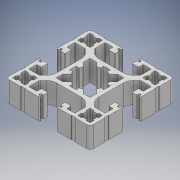
# Autodesk Inventor part: PERFIL_ESTRUTURAL_40X40_EIXO_Y_PERPENDICULAR
Saved by Autodesk Inventor 2018 (Build 220112000, 112)
## iProperties
Created: 2018-10-11
Part Number: PERFIL_ESTRUTURAL_40X40_EIXO_Y_PERPENDICULAR
Material: Genérico
Document SubType Name: Modeling
Designer: Usuario
Density: 1 g/cm^3
Appearance: Padrão
Author: Usuario
Autodesk Inventor part; units mm, degrees
ref_plane "YZ Plane" through (0, 0, 0) normal (1, 0, 0) x (0, 1, 0)
ref_plane "XZ Plane" through (0, 0, 0) normal (0, 1, 0) x (-1, 0, 0)
ref_plane "XY Plane" through (0, 0, 0) normal (0, 0, 1) x (1, 0, 0)
sketch "Esboço1" plane through (0, 0, 0) normal (0, 0, 1) x (1, 0, 0)
  arc A0 (-10, 5.8076) -> (-11.4645, 9.3431) centre (-15, 5.8076) ccw
  line L0 (-10, -5.8076) -> (-10, 5.8076)
  arc A1 (-11.4645, -9.3431) -> (-10, -5.8076) centre (-15, -5.8076) ccw
  line L1 (-12.8284, -10.7071) -> (-11.4645, -9.3431)
  arc A2 (-13.5355, -11) -> (-12.8284, -10.7071) centre (-13.5355, -10) ccw
  line L2 (-17.9, -11) -> (-13.5355, -11)
  arc A3 (-18.2, -10.7) -> (-17.9, -11) centre (-17.9, -10.7) ccw
  line L3 (-18.2, -7.45) -> (-18.2, -10.7)
  arc A4 (-17.9, -7.15) -> (-18.2, -7.45) centre (-17.9, -7.45) ccw
  line L4 (-16.3, -7.15) -> (-17.9, -7.15)
  arc A5 (-16.3, -7.15) -> (-16, -6.85) centre (-16.3, -6.85) ccw
  line L5 (-16, -4.4) -> (-16, -6.85)
  arc A6 (-16, -4.4) -> (-16.3, -4.1) centre (-16.3, -4.4) ccw
  line L6 (-17.9, -4.1) -> (-16.3, -4.1)
  arc A7 (-17.9, -4.1) -> (-18.2, -4.4) centre (-17.9, -4.4) ccw
  line L7 (-18.2, -5.05) -> (-18.2, -4.4)
  arc A8 (-18.5, -5.35) -> (-18.2, -5.05) centre (-18.5, -5.05) ccw
  line L8 (-18.9, -5.35) -> (-18.5, -5.35)
  arc A9 (-19.2, -5.05) -> (-18.9, -5.35) centre (-18.9, -5.05) ccw
  line L9 (-19.2, -4.4) -> (-19.2, -5.05)
  arc A10 (-19.2, -4.4) -> (-19.5, -4.1) centre (-19.5, -4.4) ccw
  line L10 (-19.7, -4.1) -> (-19.5, -4.1)
  arc A11 (-19.7, -4.1) -> (-20, -4.4) centre (-19.7, -4.4) ccw
  line L11 (-20, -11) -> (-20, -4.4)
  line L12 (-19.75, -11) -> (-20, -11)
  line L13 (-19.75, -13) -> (-19.75, -11)
  line L14 (-20, -13) -> (-19.75, -13)
  line L15 (-20, -18.5) -> (-20, -13)
  arc A12 (-20, -18.5) -> (-18.5, -20) centre (-18.5, -18.5) ccw
  line L16 (-13, -20) -> (-18.5, -20)
  line L17 (-13, -19.75) -> (-13, -20)
  line L18 (-11, -19.75) -> (-13, -19.75)
  line L19 (-11, -20) -> (-11, -19.75)
  line L20 (-4.4, -20) -> (-11, -20)
  arc A13 (-4.4, -20) -> (-4.1, -19.7) centre (-4.4, -19.7) ccw
  line L21 (-4.1, -19.5) -> (-4.1, -19.7)
  arc A14 (-4.1, -19.5) -> (-4.4, -19.2) centre (-4.4, -19.5) ccw
  line L22 (-5.05, -19.2) -> (-4.4, -19.2)
  arc A15 (-5.35, -18.9) -> (-5.05, -19.2) centre (-5.05, -18.9) ccw
  line L23 (-5.35, -18.5) -> (-5.35, -18.9)
  arc A16 (-5.05, -18.2) -> (-5.35, -18.5) centre (-5.05, -18.5) ccw
  line L24 (-4.4, -18.2) -> (-5.05, -18.2)
  arc A17 (-4.4, -18.2) -> (-4.1, -17.9) centre (-4.4, -17.9) ccw
  line L25 (-4.1, -16.3) -> (-4.1, -17.9)
  arc A18 (-4.1, -16.3) -> (-4.4, -16) centre (-4.4, -16.3) ccw
  line L26 (-6.85, -16) -> (-4.4, -16)
  arc A19 (-6.85, -16) -> (-7.15, -16.3) centre (-6.85, -16.3) ccw
  line L27 (-7.15, -17.9) -> (-7.15, -16.3)
  arc A20 (-7.45, -18.2) -> (-7.15, -17.9) centre (-7.45, -17.9) ccw
  line L28 (-10.7, -18.2) -> (-7.45, -18.2)
  arc A21 (-11, -17.9) -> (-10.7, -18.2) centre (-10.7, -17.9) ccw
  line L29 (-11, -13.5355) -> (-11, -17.9)
  arc A22 (-10.7071, -12.8284) -> (-11, -13.5355) centre (-10, -13.5355) ccw
  line L30 (-9.3431, -11.4645) -> (-10.7071, -12.8284)
  arc A23 (-5.8076, -10) -> (-9.3431, -11.4645) centre (-5.8076, -15) ccw
  line L31 (5.8076, -10) -> (-5.8076, -10)
  arc A24 (9.3431, -11.4645) -> (5.8076, -10) centre (5.8076, -15) ccw
  line L32 (10.7071, -12.8284) -> (9.3431, -11.4645)
  arc A25 (11, -13.5355) -> (10.7071, -12.8284) centre (10, -13.5355) ccw
  line L33 (11, -17.9) -> (11, -13.5355)
  arc A26 (10.7, -18.2) -> (11, -17.9) centre (10.7, -17.9) ccw
  line L34 (7.45, -18.2) -> (10.7, -18.2)
  arc A27 (7.15, -17.9) -> (7.45, -18.2) centre (7.45, -17.9) ccw
  line L35 (7.15, -16.3) -> (7.15, -17.9)
  arc A28 (7.15, -16.3) -> (6.85, -16) centre (6.85, -16.3) ccw
  line L36 (4.4, -16) -> (6.85, -16)
  arc A29 (4.4, -16) -> (4.1, -16.3) centre (4.4, -16.3) ccw
  line L37 (4.1, -17.9) -> (4.1, -16.3)
  arc A30 (4.1, -17.9) -> (4.4, -18.2) centre (4.4, -17.9) ccw
  line L38 (5.05, -18.2) -> (4.4, -18.2)
  arc A31 (5.35, -18.5) -> (5.05, -18.2) centre (5.05, -18.5) ccw
  line L39 (5.35, -18.9) -> (5.35, -18.5)
  arc A32 (5.05, -19.2) -> (5.35, -18.9) centre (5.05, -18.9) ccw
  line L40 (4.4, -19.2) -> (5.05, -19.2)
  arc A33 (4.4, -19.2) -> (4.1, -19.5) centre (4.4, -19.5) ccw
  line L41 (4.1, -19.7) -> (4.1, -19.5)
  arc A34 (4.1, -19.7) -> (4.4, -20) centre (4.4, -19.7) ccw
  line L42 (11, -20) -> (4.4, -20)
  line L43 (11, -19.75) -> (11, -20)
  line L44 (13, -19.75) -> (11, -19.75)
  line L45 (13, -20) -> (13, -19.75)
  line L46 (18.5, -20) -> (13, -20)
  arc A35 (18.5, -20) -> (20, -18.5) centre (18.5, -18.5) ccw
  line L47 (20, -13) -> (20, -18.5)
  line L48 (19.75, -13) -> (20, -13)
  line L49 (19.75, -11) -> (19.75, -13)
  line L50 (20, -11) -> (19.75, -11)
  line L51 (20, -4.4) -> (20, -11)
  arc A36 (20, -4.4) -> (19.7, -4.1) centre (19.7, -4.4) ccw
  line L52 (19.5, -4.1) -> (19.7, -4.1)
  arc A37 (19.5, -4.1) -> (19.2, -4.4) centre (19.5, -4.4) ccw
  line L53 (19.2, -5.05) -> (19.2, -4.4)
  arc A38 (18.9, -5.35) -> (19.2, -5.05) centre (18.9, -5.05) ccw
  line L54 (18.5, -5.35) -> (18.9, -5.35)
  arc A39 (18.2, -5.05) -> (18.5, -5.35) centre (18.5, -5.05) ccw
  line L55 (18.2, -4.4) -> (18.2, -5.05)
  arc A40 (18.2, -4.4) -> (17.9, -4.1) centre (17.9, -4.4) ccw
  line L56 (16.3, -4.1) -> (17.9, -4.1)
  arc A41 (16.3, -4.1) -> (16, -4.4) centre (16.3, -4.4) ccw
  line L57 (16, -6.85) -> (16, -4.4)
  arc A42 (16, -6.85) -> (16.3, -7.15) centre (16.3, -6.85) ccw
  line L58 (17.9, -7.15) -> (16.3, -7.15)
  arc A43 (18.2, -7.45) -> (17.9, -7.15) centre (17.9, -7.45) ccw
  line L59 (18.2, -10.7) -> (18.2, -7.45)
  arc A44 (17.9, -11) -> (18.2, -10.7) centre (17.9, -10.7) ccw
  line L60 (13.5355, -11) -> (17.9, -11)
  arc A45 (12.8284, -10.7071) -> (13.5355, -11) centre (13.5355, -10) ccw
  line L61 (11.4645, -9.3431) -> (12.8284, -10.7071)
  arc A46 (10, -5.8076) -> (11.4645, -9.3431) centre (15, -5.8076) ccw
  line L62 (10, 5.8076) -> (10, -5.8076)
  arc A47 (11.4645, 9.3431) -> (10, 5.8076) centre (15, 5.8076) ccw
  line L63 (12.8284, 10.7071) -> (11.4645, 9.3431)
  arc A48 (13.5355, 11) -> (12.8284, 10.7071) centre (13.5355, 10) ccw
  line L64 (17.9, 11) -> (13.5355, 11)
  arc A49 (18.2, 10.7) -> (17.9, 11) centre (17.9, 10.7) ccw
  line L65 (18.2, 7.45) -> (18.2, 10.7)
  arc A50 (17.9, 7.15) -> (18.2, 7.45) centre (17.9, 7.45) ccw
  line L66 (16.3, 7.15) -> (17.9, 7.15)
  arc A51 (16.3, 7.15) -> (16, 6.85) centre (16.3, 6.85) ccw
  line L67 (16, 4.4) -> (16, 6.85)
  arc A52 (16, 4.4) -> (16.3, 4.1) centre (16.3, 4.4) ccw
  line L68 (17.9, 4.1) -> (16.3, 4.1)
  arc A53 (17.9, 4.1) -> (18.2, 4.4) centre (17.9, 4.4) ccw
  line L69 (18.2, 5.05) -> (18.2, 4.4)
  arc A54 (18.5, 5.35) -> (18.2, 5.05) centre (18.5, 5.05) ccw
  line L70 (18.9, 5.35) -> (18.5, 5.35)
  arc A55 (19.2, 5.05) -> (18.9, 5.35) centre (18.9, 5.05) ccw
  line L71 (19.2, 4.4) -> (19.2, 5.05)
  arc A56 (19.2, 4.4) -> (19.5, 4.1) centre (19.5, 4.4) ccw
  line L72 (19.7, 4.1) -> (19.5, 4.1)
  arc A57 (19.7, 4.1) -> (20, 4.4) centre (19.7, 4.4) ccw
  line L73 (20, 11) -> (20, 4.4)
  line L74 (19.75, 11) -> (20, 11)
  line L75 (19.75, 13) -> (19.75, 11)
  line L76 (20, 13) -> (19.75, 13)
  line L77 (20, 18.5) -> (20, 13)
  arc A58 (20, 18.5) -> (18.5, 20) centre (18.5, 18.5) ccw
  line L78 (13, 20) -> (18.5, 20)
  line L79 (13, 19.75) -> (13, 20)
  line L80 (11, 19.75) -> (13, 19.75)
  line L81 (11, 20) -> (11, 19.75)
  line L82 (4.4, 20) -> (11, 20)
  arc A59 (4.4, 20) -> (4.1, 19.7) centre (4.4, 19.7) ccw
  line L83 (4.1, 19.5) -> (4.1, 19.7)
  arc A60 (4.1, 19.5) -> (4.4, 19.2) centre (4.4, 19.5) ccw
  line L84 (5.05, 19.2) -> (4.4, 19.2)
  arc A61 (5.35, 18.9) -> (5.05, 19.2) centre (5.05, 18.9) ccw
  line L85 (5.35, 18.5) -> (5.35, 18.9)
  arc A62 (5.05, 18.2) -> (5.35, 18.5) centre (5.05, 18.5) ccw
  line L86 (4.4, 18.2) -> (5.05, 18.2)
  arc A63 (4.4, 18.2) -> (4.1, 17.9) centre (4.4, 17.9) ccw
  line L87 (4.1, 16.3) -> (4.1, 17.9)
  arc A64 (4.1, 16.3) -> (4.4, 16) centre (4.4, 16.3) ccw
  line L88 (6.85, 16) -> (4.4, 16)
  arc A65 (6.85, 16) -> (7.15, 16.3) centre (6.85, 16.3) ccw
  line L89 (7.15, 17.9) -> (7.15, 16.3)
  arc A66 (7.45, 18.2) -> (7.15, 17.9) centre (7.45, 17.9) ccw
  line L90 (10.7, 18.2) -> (7.45, 18.2)
  arc A67 (11, 17.9) -> (10.7, 18.2) centre (10.7, 17.9) ccw
  line L91 (11, 13.5355) -> (11, 17.9)
  arc A68 (10.7071, 12.8284) -> (11, 13.5355) centre (10, 13.5355) ccw
  line L92 (9.3431, 11.4645) -> (10.7071, 12.8284)
  arc A69 (5.8076, 10) -> (9.3431, 11.4645) centre (5.8076, 15) ccw
  line L93 (-5.8076, 10) -> (5.8076, 10)
  arc A70 (-9.3431, 11.4645) -> (-5.8076, 10) centre (-5.8076, 15) ccw
  line L94 (-10.7071, 12.8284) -> (-9.3431, 11.4645)
  arc A71 (-11, 13.5355) -> (-10.7071, 12.8284) centre (-10, 13.5355) ccw
  line L95 (-11, 17.9) -> (-11, 13.5355)
  arc A72 (-10.7, 18.2) -> (-11, 17.9) centre (-10.7, 17.9) ccw
  line L96 (-7.45, 18.2) -> (-10.7, 18.2)
  arc A73 (-7.15, 17.9) -> (-7.45, 18.2) centre (-7.45, 17.9) ccw
  line L97 (-7.15, 16.3) -> (-7.15, 17.9)
  arc A74 (-7.15, 16.3) -> (-6.85, 16) centre (-6.85, 16.3) ccw
  line L98 (-4.4, 16) -> (-6.85, 16)
  arc A75 (-4.4, 16) -> (-4.1, 16.3) centre (-4.4, 16.3) ccw
  line L99 (-4.1, 17.9) -> (-4.1, 16.3)
  arc A76 (-4.1, 17.9) -> (-4.4, 18.2) centre (-4.4, 17.9) ccw
  line L100 (-5.05, 18.2) -> (-4.4, 18.2)
  arc A77 (-5.35, 18.5) -> (-5.05, 18.2) centre (-5.05, 18.5) ccw
  line L101 (-5.35, 18.9) -> (-5.35, 18.5)
  arc A78 (-5.05, 19.2) -> (-5.35, 18.9) centre (-5.05, 18.9) ccw
  line L102 (-4.4, 19.2) -> (-5.05, 19.2)
  arc A79 (-4.4, 19.2) -> (-4.1, 19.5) centre (-4.4, 19.5) ccw
  line L103 (-4.1, 19.7) -> (-4.1, 19.5)
  arc A80 (-4.1, 19.7) -> (-4.4, 20) centre (-4.4, 19.7) ccw
  line L104 (-11, 20) -> (-4.4, 20)
  line L105 (-11, 19.75) -> (-11, 20)
  line L106 (-13, 19.75) -> (-11, 19.75)
  line L107 (-13, 20) -> (-13, 19.75)
  line L108 (-18.5, 20) -> (-13, 20)
  arc A81 (-18.5, 20) -> (-20, 18.5) centre (-18.5, 18.5) ccw
  line L109 (-20, 13) -> (-20, 18.5)
  line L110 (-19.75, 13) -> (-20, 13)
  line L111 (-19.75, 11) -> (-19.75, 13)
  line L112 (-20, 11) -> (-19.75, 11)
  line L113 (-20, 4.4) -> (-20, 11)
  arc A82 (-20, 4.4) -> (-19.7, 4.1) centre (-19.7, 4.4) ccw
  line L114 (-19.5, 4.1) -> (-19.7, 4.1)
  arc A83 (-19.5, 4.1) -> (-19.2, 4.4) centre (-19.5, 4.4) ccw
  line L115 (-19.2, 5.05) -> (-19.2, 4.4)
  arc A84 (-18.9, 5.35) -> (-19.2, 5.05) centre (-18.9, 5.05) ccw
  line L116 (-18.5, 5.35) -> (-18.9, 5.35)
  arc A85 (-18.2, 5.05) -> (-18.5, 5.35) centre (-18.5, 5.05) ccw
  line L117 (-18.2, 4.4) -> (-18.2, 5.05)
  arc A86 (-18.2, 4.4) -> (-17.9, 4.1) centre (-17.9, 4.4) ccw
  line L118 (-16.3, 4.1) -> (-17.9, 4.1)
  arc A87 (-16.3, 4.1) -> (-16, 4.4) centre (-16.3, 4.4) ccw
  line L119 (-16, 6.85) -> (-16, 4.4)
  arc A88 (-16, 6.85) -> (-16.3, 7.15) centre (-16.3, 6.85) ccw
  line L120 (-17.9, 7.15) -> (-16.3, 7.15)
  arc A89 (-18.2, 7.45) -> (-17.9, 7.15) centre (-17.9, 7.45) ccw
  line L121 (-18.2, 10.7) -> (-18.2, 7.45)
  arc A90 (-17.9, 11) -> (-18.2, 10.7) centre (-17.9, 10.7) ccw
  line L122 (-13.5355, 11) -> (-17.9, 11)
  arc A91 (-12.8284, 10.7071) -> (-13.5355, 11) centre (-13.5355, 10) ccw
  line L123 (-11.4645, 9.3431) -> (-12.8284, 10.7071)
  arc A92 (16.5, -18.2) -> (16.8, -18.5) centre (16.8, -18.2) ccw
  line L124 (16.5, -18.2) -> (16.5, -17.7913)
  arc A93 (14.5, -17.7913) -> (16.5, -17.7913) centre (15.5, -15.5) ccw
  line L125 (14.5, -17.7913) -> (14.5, -18.2)
  arc A94 (14.2, -18.5) -> (14.5, -18.2) centre (14.2, -18.2) ccw
  line L126 (14.2, -18.5) -> (12.8, -18.5)
  arc A95 (12.5, -18.2) -> (12.8, -18.5) centre (12.8, -18.2) ccw
  line L127 (12.5, -18.2) -> (12.5, -16.8)
  arc A96 (12.8, -16.5) -> (12.5, -16.8) centre (12.8, -16.8) ccw
  line L128 (12.8, -16.5) -> (13.2087, -16.5)
  arc A97 (13.2087, -14.5) -> (13.2087, -16.5) centre (15.5, -15.5) ccw
  line L129 (13.2087, -14.5) -> (12.8, -14.5)
  arc A98 (12.5, -14.2) -> (12.8, -14.5) centre (12.8, -14.2) ccw
  line L130 (12.5, -14.2) -> (12.5, -12.8)
  arc A99 (12.8, -12.5) -> (12.5, -12.8) centre (12.8, -12.8) ccw
  line L131 (12.8, -12.5) -> (14.2, -12.5)
  arc A100 (14.5, -12.8) -> (14.2, -12.5) centre (14.2, -12.8) ccw
  line L132 (14.5, -12.8) -> (14.5, -13.2087)
  arc A101 (16.5, -13.2087) -> (14.5, -13.2087) centre (15.5, -15.5) ccw
  line L133 (16.5, -13.2087) -> (16.5, -12.8)
  arc A102 (16.8, -12.5) -> (16.5, -12.8) centre (16.8, -12.8) ccw
  line L134 (16.8, -12.5) -> (18.2, -12.5)
  arc A103 (18.5, -12.8) -> (18.2, -12.5) centre (18.2, -12.8) ccw
  line L135 (18.5, -12.8) -> (18.5, -14.2)
  arc A104 (18.2, -14.5) -> (18.5, -14.2) centre (18.2, -14.2) ccw
  line L136 (18.2, -14.5) -> (17.7913, -14.5)
  arc A105 (17.7913, -16.5) -> (17.7913, -14.5) centre (15.5, -15.5) ccw
  line L137 (17.7913, -16.5) -> (18.2, -16.5)
  arc A106 (18.5, -16.8) -> (18.2, -16.5) centre (18.2, -16.8) ccw
  line L138 (18.5, -16.8) -> (18.5, -18.2)
  arc A107 (18.2, -18.5) -> (18.5, -18.2) centre (18.2, -18.2) ccw
  line L139 (18.2, -18.5) -> (16.8, -18.5)
  arc A108 (-1.6602, 6.6458) -> (-1.4391, 6.9972) centre (-1.7329, 6.9368) ccw
  line L140 (-1.4391, 6.9972) -> (-1.662, 8.0809)
  arc A109 (1.662, 8.0809) -> (-1.662, 8.0809) centre (0, 0) ccw
  line L141 (1.662, 8.0809) -> (1.4391, 6.9972)
  arc A110 (1.4391, 6.9972) -> (1.6602, 6.6458) centre (1.7329, 6.9368) ccw
  arc A111 (2.7977, 6.2526) -> (1.6602, 6.6458) centre (0, 0) ccw
  arc A112 (2.7977, 6.2526) -> (3.1324, 6.3143) centre (2.9202, 6.5265) ccw
  line L142 (3.1324, 6.3143) -> (4.8891, 8.0711)
  line L143 (4.8891, 8.0711) -> (8.0711, 8.0711)
  line L144 (8.0711, 8.0711) -> (8.0711, 4.8891)
  line L145 (8.0711, 4.8891) -> (6.3143, 3.1324)
  arc A113 (6.3143, 3.1324) -> (6.2526, 2.7977) centre (6.5265, 2.9202) ccw
  arc A114 (6.6458, 1.6602) -> (6.2526, 2.7977) centre (0, 0) ccw
  arc A115 (6.6458, 1.6602) -> (6.9972, 1.4391) centre (6.9368, 1.7329) ccw
  line L146 (6.9972, 1.4391) -> (8.0809, 1.662)
  arc A116 (8.0809, -1.662) -> (8.0809, 1.662) centre (0, 0) ccw
  line L147 (8.0809, -1.662) -> (6.9972, -1.4391)
  arc A117 (6.9972, -1.4391) -> (6.6458, -1.6602) centre (6.9368, -1.7329) ccw
  arc A118 (6.2526, -2.7977) -> (6.6458, -1.6602) centre (0, 0) ccw
  arc A119 (6.2526, -2.7977) -> (6.3143, -3.1324) centre (6.5265, -2.9202) ccw
  line L148 (6.3143, -3.1324) -> (8.0711, -4.8891)
  line L149 (8.0711, -4.8891) -> (8.0711, -8.0711)
  line L150 (8.0711, -8.0711) -> (4.8891, -8.0711)
  line L151 (4.8891, -8.0711) -> (3.1324, -6.3143)
  arc A120 (3.1324, -6.3143) -> (2.7977, -6.2526) centre (2.9202, -6.5265) ccw
  arc A121 (1.6602, -6.6458) -> (2.7977, -6.2526) centre (0, 0) ccw
  arc A122 (1.6602, -6.6458) -> (1.4391, -6.9972) centre (1.7329, -6.9368) ccw
  line L152 (1.4391, -6.9972) -> (1.662, -8.0809)
  arc A123 (-1.662, -8.0809) -> (1.662, -8.0809) centre (0, 0) ccw
  line L153 (-1.662, -8.0809) -> (-1.4391, -6.9972)
  arc A124 (-1.4391, -6.9972) -> (-1.6602, -6.6458) centre (-1.7329, -6.9368) ccw
  arc A125 (-2.7977, -6.2526) -> (-1.6602, -6.6458) centre (0, 0) ccw
  arc A126 (-2.7977, -6.2526) -> (-3.1324, -6.3143) centre (-2.9202, -6.5265) ccw
  line L154 (-3.1324, -6.3143) -> (-4.8891, -8.0711)
  line L155 (-4.8891, -8.0711) -> (-8.0711, -8.0711)
  line L156 (-8.0711, -8.0711) -> (-8.0711, -4.8891)
  line L157 (-8.0711, -4.8891) -> (-6.3143, -3.1324)
  arc A127 (-6.3143, -3.1324) -> (-6.2526, -2.7977) centre (-6.5265, -2.9202) ccw
  arc A128 (-6.6458, -1.6602) -> (-6.2526, -2.7977) centre (0, 0) ccw
  arc A129 (-6.6458, -1.6602) -> (-6.9972, -1.4391) centre (-6.9368, -1.7329) ccw
  line L158 (-6.9972, -1.4391) -> (-8.0809, -1.662)
  arc A130 (-8.0809, 1.662) -> (-8.0809, -1.662) centre (0, 0) ccw
  line L159 (-8.0809, 1.662) -> (-6.9972, 1.4391)
  arc A131 (-6.9972, 1.4391) -> (-6.6458, 1.6602) centre (-6.9368, 1.7329) ccw
  arc A132 (-6.2526, 2.7977) -> (-6.6458, 1.6602) centre (0, 0) ccw
  arc A133 (-6.2526, 2.7977) -> (-6.3143, 3.1324) centre (-6.5265, 2.9202) ccw
  line L160 (-6.3143, 3.1324) -> (-8.0711, 4.8891)
  line L161 (-8.0711, 4.8891) -> (-8.0711, 8.0711)
  line L162 (-8.0711, 8.0711) -> (-4.8891, 8.0711)
  line L163 (-4.8891, 8.0711) -> (-3.1324, 6.3143)
  arc A134 (-3.1324, 6.3143) -> (-2.7977, 6.2526) centre (-2.9202, 6.5265) ccw
  arc A135 (-1.6602, 6.6458) -> (-2.7977, 6.2526) centre (0, 0) ccw
  arc A136 (-17.7913, 16.5) -> (-17.7913, 14.5) centre (-15.5, 15.5) ccw
  line L164 (-17.7913, 16.5) -> (-18.2, 16.5)
  arc A137 (-18.5, 16.8) -> (-18.2, 16.5) centre (-18.2, 16.8) ccw
  line L165 (-18.5, 16.8) -> (-18.5, 18.2)
  arc A138 (-18.2, 18.5) -> (-18.5, 18.2) centre (-18.2, 18.2) ccw
  line L166 (-18.2, 18.5) -> (-16.8, 18.5)
  arc A139 (-16.5, 18.2) -> (-16.8, 18.5) centre (-16.8, 18.2) ccw
  line L167 (-16.5, 18.2) -> (-16.5, 17.7913)
  arc A140 (-14.5, 17.7913) -> (-16.5, 17.7913) centre (-15.5, 15.5) ccw
  line L168 (-14.5, 17.7913) -> (-14.5, 18.2)
  arc A141 (-14.2, 18.5) -> (-14.5, 18.2) centre (-14.2, 18.2) ccw
  line L169 (-14.2, 18.5) -> (-12.8, 18.5)
  arc A142 (-12.5, 18.2) -> (-12.8, 18.5) centre (-12.8, 18.2) ccw
  line L170 (-12.5, 18.2) -> (-12.5, 16.8)
  arc A143 (-12.8, 16.5) -> (-12.5, 16.8) centre (-12.8, 16.8) ccw
  line L171 (-12.8, 16.5) -> (-13.2087, 16.5)
  arc A144 (-13.2087, 14.5) -> (-13.2087, 16.5) centre (-15.5, 15.5) ccw
  line L172 (-13.2087, 14.5) -> (-12.8, 14.5)
  arc A145 (-12.5, 14.2) -> (-12.8, 14.5) centre (-12.8, 14.2) ccw
  line L173 (-12.5, 14.2) -> (-12.5, 12.8)
  arc A146 (-12.8, 12.5) -> (-12.5, 12.8) centre (-12.8, 12.8) ccw
  line L174 (-12.8, 12.5) -> (-14.2, 12.5)
  arc A147 (-14.5, 12.8) -> (-14.2, 12.5) centre (-14.2, 12.8) ccw
  line L175 (-14.5, 12.8) -> (-14.5, 13.2087)
  arc A148 (-16.5, 13.2087) -> (-14.5, 13.2087) centre (-15.5, 15.5) ccw
  line L176 (-16.5, 13.2087) -> (-16.5, 12.8)
  arc A149 (-16.8, 12.5) -> (-16.5, 12.8) centre (-16.8, 12.8) ccw
  line L177 (-16.8, 12.5) -> (-18.2, 12.5)
  arc A150 (-18.5, 12.8) -> (-18.2, 12.5) centre (-18.2, 12.8) ccw
  line L178 (-18.5, 12.8) -> (-18.5, 14.2)
  arc A151 (-18.2, 14.5) -> (-18.5, 14.2) centre (-18.2, 14.2) ccw
  line L179 (-18.2, 14.5) -> (-17.7913, 14.5)
  arc A152 (-17.7913, -14.5) -> (-17.7913, -16.5) centre (-15.5, -15.5) ccw
  line L180 (-17.7913, -14.5) -> (-18.2, -14.5)
  arc A153 (-18.5, -14.2) -> (-18.2, -14.5) centre (-18.2, -14.2) ccw
  line L181 (-18.5, -14.2) -> (-18.5, -12.8)
  arc A154 (-18.2, -12.5) -> (-18.5, -12.8) centre (-18.2, -12.8) ccw
  line L182 (-18.2, -12.5) -> (-16.8, -12.5)
  arc A155 (-16.5, -12.8) -> (-16.8, -12.5) centre (-16.8, -12.8) ccw
  line L183 (-16.5, -12.8) -> (-16.5, -13.2087)
  arc A156 (-14.5, -13.2087) -> (-16.5, -13.2087) centre (-15.5, -15.5) ccw
  line L184 (-14.5, -13.2087) -> (-14.5, -12.8)
  arc A157 (-14.2, -12.5) -> (-14.5, -12.8) centre (-14.2, -12.8) ccw
  line L185 (-14.2, -12.5) -> (-12.8, -12.5)
  arc A158 (-12.5, -12.8) -> (-12.8, -12.5) centre (-12.8, -12.8) ccw
  line L186 (-12.5, -12.8) -> (-12.5, -14.2)
  arc A159 (-12.8, -14.5) -> (-12.5, -14.2) centre (-12.8, -14.2) ccw
  line L187 (-12.8, -14.5) -> (-13.2087, -14.5)
  arc A160 (-13.2087, -16.5) -> (-13.2087, -14.5) centre (-15.5, -15.5) ccw
  line L188 (-13.2087, -16.5) -> (-12.8, -16.5)
  arc A161 (-12.5, -16.8) -> (-12.8, -16.5) centre (-12.8, -16.8) ccw
  line L189 (-12.5, -16.8) -> (-12.5, -18.2)
  arc A162 (-12.8, -18.5) -> (-12.5, -18.2) centre (-12.8, -18.2) ccw
  line L190 (-12.8, -18.5) -> (-14.2, -18.5)
  arc A163 (-14.5, -18.2) -> (-14.2, -18.5) centre (-14.2, -18.2) ccw
  line L191 (-14.5, -18.2) -> (-14.5, -17.7913)
  arc A164 (-16.5, -17.7913) -> (-14.5, -17.7913) centre (-15.5, -15.5) ccw
  line L192 (-16.5, -17.7913) -> (-16.5, -18.2)
  arc A165 (-16.8, -18.5) -> (-16.5, -18.2) centre (-16.8, -18.2) ccw
  line L193 (-16.8, -18.5) -> (-18.2, -18.5)
  arc A166 (-18.5, -18.2) -> (-18.2, -18.5) centre (-18.2, -18.2) ccw
  line L194 (-18.5, -18.2) -> (-18.5, -16.8)
  arc A167 (-18.2, -16.5) -> (-18.5, -16.8) centre (-18.2, -16.8) ccw
  line L195 (-18.2, -16.5) -> (-17.7913, -16.5)
  arc A168 (17.7913, 14.5) -> (17.7913, 16.5) centre (15.5, 15.5) ccw
  line L196 (17.7913, 14.5) -> (18.2, 14.5)
  arc A169 (18.5, 14.2) -> (18.2, 14.5) centre (18.2, 14.2) ccw
  line L197 (18.5, 14.2) -> (18.5, 12.8)
  arc A170 (18.2, 12.5) -> (18.5, 12.8) centre (18.2, 12.8) ccw
  line L198 (18.2, 12.5) -> (16.8, 12.5)
  arc A171 (16.5, 12.8) -> (16.8, 12.5) centre (16.8, 12.8) ccw
  line L199 (16.5, 12.8) -> (16.5, 13.2087)
  arc A172 (14.5, 13.2087) -> (16.5, 13.2087) centre (15.5, 15.5) ccw
  line L200 (14.5, 13.2087) -> (14.5, 12.8)
  arc A173 (14.2, 12.5) -> (14.5, 12.8) centre (14.2, 12.8) ccw
  line L201 (14.2, 12.5) -> (12.8, 12.5)
  arc A174 (12.5, 12.8) -> (12.8, 12.5) centre (12.8, 12.8) ccw
  line L202 (12.5, 12.8) -> (12.5, 14.2)
  arc A175 (12.8, 14.5) -> (12.5, 14.2) centre (12.8, 14.2) ccw
  line L203 (12.8, 14.5) -> (13.2087, 14.5)
  arc A176 (13.2087, 16.5) -> (13.2087, 14.5) centre (15.5, 15.5) ccw
  line L204 (13.2087, 16.5) -> (12.8, 16.5)
  arc A177 (12.5, 16.8) -> (12.8, 16.5) centre (12.8, 16.8) ccw
  line L205 (12.5, 16.8) -> (12.5, 18.2)
  arc A178 (12.8, 18.5) -> (12.5, 18.2) centre (12.8, 18.2) ccw
  line L206 (12.8, 18.5) -> (14.2, 18.5)
  arc A179 (14.5, 18.2) -> (14.2, 18.5) centre (14.2, 18.2) ccw
  line L207 (14.5, 18.2) -> (14.5, 17.7913)
  arc A180 (16.5, 17.7913) -> (14.5, 17.7913) centre (15.5, 15.5) ccw
  line L208 (16.5, 17.7913) -> (16.5, 18.2)
  arc A181 (16.8, 18.5) -> (16.5, 18.2) centre (16.8, 18.2) ccw
  line L209 (16.8, 18.5) -> (18.2, 18.5)
  arc A182 (18.5, 18.2) -> (18.2, 18.5) centre (18.2, 18.2) ccw
  line L210 (18.5, 18.2) -> (18.5, 16.8)
  arc A183 (18.2, 16.5) -> (18.5, 16.8) centre (18.2, 16.8) ccw
  line L211 (18.2, 16.5) -> (17.7913, 16.5)
  constraints: 424 end point, 368 point on circle, 184 centre point
extrude "Extrusão1" add sketch "Esboço1" along normal blind 10
